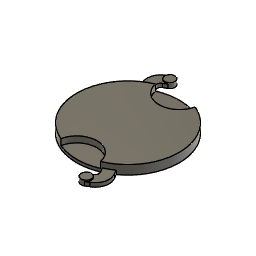
Deckbox - Assembled (Autodesk Fusion 360 archive; units mm, degrees)
design "Deckbox - Key"
Autodesk Fusion 360 part; units mm, degrees
sketch "Sketch1" plane through (0, 0, 0) normal (0, 1, 0) x (1, 0, 0)
  circle A0 centre (0, 0) radius 25.4
  line L0 (19.5918, -28.934) -> (-15.2617, 31.434)
  line L1 (-19.5918, 28.934) -> (15.2617, -31.434)
  line L2 (0, -25.4) -> (0, 25.4) construction
  line L3 (0, 0) -> (25.4, 0) construction
  line L4 (-19.5918, 28.934) -> (-15.2617, 31.434)
  line L5 (15.2617, -31.434) -> (19.5918, -28.934)
  line L6 (17.4268, -30.184) -> (-17.4268, 30.184) construction
  line L7 (-2.1651, -1.25) -> (2.1651, 1.25) construction
  line L8 (19.5918, -28.934) -> (11.7976, -33.434)
  line L9 (11.7976, -33.434) -> (9.2976, -29.1039)
  line L10 (9.2976, -29.1039) -> (17.0918, -24.6039)
  line L11 (17.0918, -24.6039) -> (19.5918, -28.934)
  circle A1 centre (10.5476, -31.269) radius 2.5
  circle A2 centre (0, 0) radius 35.5
  line L12 (-19.5918, 28.934) -> (-17.0918, 24.6039)
  line L13 (-17.0918, 24.6039) -> (-9.2976, 29.1039)
  line L14 (-9.2976, 29.1039) -> (-11.7976, 33.434)
  line L15 (-11.7976, 33.434) -> (-19.5918, 28.934)
  circle A3 centre (-10.5476, 31.269) radius 2.5
  point P0 (-12.5, 21.6506)
  point P1 (12.5, -21.6506)
  dimension "d1" = 50.8
  dimension "d42" = 5
  dimension "d45" = 5
  dimension "d46" = 71
  dimension "d47" = 60
  dimension "d48" = 4
  dimension "d51" = 5
  constraint coincident A0.centre L3.start
  constraint coincident A0 L2.start
  constraint coincident A0 L2.end
  constraint coincident A0.centre L2
  constraint coincident A0 L3.end
  constraint horizontal L3
  constraint perpendicular L0 L4
  constraint perpendicular L0 L5
  constraint perpendicular L1 L4
  constraint midpoint L5 L6.start
  constraint midpoint L4 L6.end
  constraint perpendicular L4 L6
  constraint midpoint L1 L7.start
  constraint midpoint L0 L7.end
  constraint midpoint L6 A0.centre
  constraint perpendicular L8 L9
  constraint parallel L8 L10
  constraint parallel L9 L11
  constraint perpendicular L0 L8
  constraint midpoint L9 A1.centre
  constraint tangent L10 A1
  constraint concentric A0 A2
  constraint tangent A1 A2
  constraint perpendicular L12 L13
  constraint parallel L12 L14
  constraint parallel L13 L15
  constraint coincident L1 L12.end
  constraint midpoint L14 A3.centre
  constraint tangent L13 A3
  constraint tangent A2 A3
  measures "d1" diameter of A0
  measures "d42" distance of L0 L1
  measures "d45" diameter of A1
  measures "d46" diameter of A2 A0.centre
  measures "d47" angle of L3 L6
  measures "d48" distance of L1 A1.centre
  measures "d51" diameter of A3
extrude "Extrude1" add sketch "Sketch1" along normal blind 4.5 contours A0 L0 | A0 L0 L1 | A0 L1
extrude "Extrude2" add sketch "Sketch1" along normal blind 1.9 contours A0 L0 | A0 L0 L1 | A0 L0 L1 L13 | A0 L0 L1 L10 | A0 L1 | L0 L1 L4 L12 L13 L15 | L0 L13 L15 A3 | L0 L1 L5 L8 L10 L11 | L14 A3 | L14 A3 | L1 L8 L10 A1 | L9 A1 | L9 A1
extrude "Extrude3" add sketch "Sketch1" along normal blind 2.5 contours L14 A3 | L14 A3 | L9 A1 | L9 A1
sketch "Sketch2" plane through (0, 4.5, 0) normal (0, 1, 0) x (-1, 0, 0)
  circle A0 centre (0, 0) radius 25.4
  circle A1 centre (0, -25.4) radius 10
  circle A2 centre (0, 25.4) radius 10
  line L0 (0, -25.4) -> (0, 25.4) construction
  dimension "d18" = 20
  dimension "d19" = 20
  constraint coincident A0 A1.centre
  constraint coincident A0 A2.centre
  constraint coincident A1.centre L0.start
  constraint coincident A2.centre L0.end
  constraint coincident A0.centre L0
  constraint vertical L0
  measures "d18" diameter of A1
  measures "d19" diameter of A2
extrude "Extrude4" cut sketch "Sketch2" against normal blind 3 contours A0 A2 | A0 A1 picked at (-1.832, 22.0709) picked at (1.832, -22.0709)
fillet "Fillet6" radius 2 2 edges at (12.7617, 0.95, 27.1039) (-12.7617, 0.95, -27.1039)
fillet "Fillet7" radius 7 2 edges at (19.5918, 0.95, 28.934) (-19.5918, 0.95, -28.934)
named bodies: "Deckbox - Key"

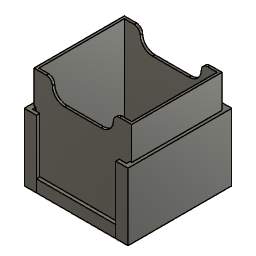
design "Deckbox - Base"
Autodesk Fusion 360 part; units mm, degrees
sketch "Sketch1" plane through (0, 0, 0) normal (0, 1, 0) x (1, 0, 0)
  line L0 (0, 0) -> (76, 0)
  line L1 (76, 0) -> (76, 70)
  line L2 (76, 70) -> (0, 70)
  line L3 (0, 70) -> (0, 0)
  line L4 (-2.25, -2.25) -> (78.25, -2.25)
  line L5 (78.25, -2.25) -> (78.25, 72.25)
  line L6 (78.25, 72.25) -> (-2.25, 72.25)
  line L7 (-2.25, 72.25) -> (-2.25, -2.25)
  line L8 (-0.5, -2.25) -> (76.5, -2.25)
  line L9 (76.5, -2.25) -> (76.5, -4.75)
  line L10 (76.5, -4.75) -> (-0.5, -4.75)
  line L11 (-0.5, -4.75) -> (-0.5, -2.25)
  line L12 (-0.5, -2.25) -> (-4.5, -2.25)
  line L13 (-4.5, -2.25) -> (-4.5, -7.5)
  line L14 (-4.5, -7.5) -> (5.5, -7.5)
  line L15 (5.5, -7.5) -> (5.5, -4.75)
  line L16 (76.5, -2.25) -> (80.5, -2.25)
  line L17 (80.5, -2.25) -> (80.5, -7.5)
  line L18 (80.5, -7.5) -> (70.5, -7.5)
  line L19 (70.5, -7.5) -> (70.5, -4.75)
  line L20 (-4.5, -2.25) -> (80.5, -2.25)
  line L21 (80.5, -2.25) -> (80.5, 77.5)
  line L22 (80.5, 77.5) -> (-4.5, 77.5)
  line L23 (-4.5, 77.5) -> (-4.5, -2.25)
  line L24 (5.5, -7.5) -> (70.5, -7.5)
  point P0 (38, -2.25)
  point P1 (38, -2.25)
  dimension "d3" = 2.25
  dimension "d5" = 2.25
  dimension "d6" = 2.25
  dimension "d7" = 2.25
  dimension "d19" = 77
  dimension "d27" = 10
  dimension "d29" = 5.25
  dimension "d30" = 2.25
  dimension "d58" = 5.25
  dimension "d59" = 2.5
  dimension "d61" = 10
  dimension "d62" = 2.25
  dimension "d77" = 85
  dimension "d78" = 85
  constraint horizontal L0
  constraint vertical L1
  constraint horizontal L2
  constraint vertical L3
  constraint coincident L0.start L3.end
  constraint horizontal L4
  constraint vertical L5
  constraint horizontal L6
  constraint vertical L7
  constraint horizontal L8
  constraint vertical L9
  constraint horizontal L10
  constraint vertical L11
  constraint perpendicular L11 L12
  constraint perpendicular L12 L13
  constraint perpendicular L13 L14
  constraint coincident L10 L15.end
  constraint perpendicular L10 L15
  constraint perpendicular L9 L16
  constraint perpendicular L16 L17
  constraint perpendicular L17 L18
  constraint coincident L10 L19.end
  constraint perpendicular L10 L19
  constraint midpoint L8 P1
  constraint midpoint L4 P1
  constraint coincident P1 P0
  constraint horizontal L20
  constraint vertical L21
  constraint horizontal L22
  constraint vertical L23
  constraint coincident L17 L16.end
  constraint horizontal L24
  measures "d3" distance of L1 L5
  measures "d5" distance of L2 L6
  measures "d6" distance of L3 L7
  measures "d7" distance of L0 L4
  measures "d19" distance of L8.start L8.end
  measures "d27" distance of L17 L19
  measures "d29" distance of L6 L22
  measures "d30" distance of L5 L21
  measures "d58" distance of L4 L24
  measures "d59" distance of L10 L20
  measures "d61" distance of L13 L15
  measures "d62" distance of L7 L23
  measures "d77" distance of L13.end L17.end L0.start
  measures "d78" distance of L13.end L22.end
extrude "Extrude1" add sketch "Sketch1" against normal blind 2 contours L0 L1 L2 L3 | L4 L5 L6 L7 L8 L12 L16 L20 | L5 L6 L7 L12 L16 L20 L21 L22 L23 | L4 L10 L11 L12 L13 L14 L15 L20 | L4 L8 L9 L10 L11 L20 | L4 L9 L10 L16 L17 L18 L19 L20 | L10 L15 L19 L24
extrude "Extrude2" add sketch "Sketch1" along normal blind 80 contours L4 L5 L6 L7 L8 L12 L16 L20
extrude "Extrude3" add sketch "Sketch1" along normal blind 53 contours L5 L6 L7 L12 L16 L20 L21 L22 L23 | L4 L10 L11 L12 L13 L14 L15 L20 | L4 L9 L10 L16 L17 L18 L19 L20
extrude "Extrude5" add sketch "Sketch1" along normal blind 8 contours L10 L15 L19 L24
sketch "Sketch8" plane through (0, 80, 0) normal (0, 1, 0) x (-1, 0, 0)
  line L0 (-78.25, -72.25) -> (2.25, -72.25)
  line L1 (2.25, -72.25) -> (2.25, 2.25)
  line L2 (2.25, 2.25) -> (-78.25, 2.25)
  line L3 (-76, 0) -> (0, 0)
  line L4 (0, 0) -> (0, -70)
  line L5 (0, -70) -> (-76, -70)
  line L6 (2.25, -72.25) -> (-78.25, -72.25)
  line L7 (-78.25, -72.25) -> (-78.25, 2.25)
  line L8 (-78.25, 2.25) -> (2.25, 2.25)
  line L9 (2.25, 2.25) -> (2.25, -72.25)
  line L10 (2, -72) -> (-78, -72)
  line L11 (-78, -72) -> (-78, 2)
  line L12 (-78, 2) -> (2, 2)
  line L13 (2, 2) -> (2, -72)
  line L14 (0.5, 2.25) -> (0.5, 2)
  line L15 (-76.5, 2.25) -> (-76.5, 2)
  line L16 (0.5, 4.75) -> (0.5, 2.25)
  line L17 (-76.5, 2.25) -> (-76.5, 4.75)
  line L18 (-76, -70) -> (-76, 0)
  line L19 (-78.25, 2.25) -> (-78.25, -72.25)
  point P0 (-78.25, 2.25)
  dimension "d80" = 0.25
  dimension "d81" = 0.25
  dimension "d82" = 0.25
  dimension "d83" = 0.25
  constraint horizontal L6
  constraint vertical L7
  constraint horizontal L8
  constraint vertical L9
  constraint coincident L0.end L1.start
  constraint coincident L1.end L2.start
  constraint coincident P0 L2.end
  constraint horizontal L10
  constraint vertical L11
  constraint horizontal L12
  constraint vertical L13
  constraint coincident L12 L14.end
  constraint perpendicular L12 L14
  constraint coincident L12 L15.end
  constraint perpendicular L12 L15
  constraint coincident L8 L14.start
  constraint coincident L14.start L16
  constraint coincident L15.start L17
  measures "d80" distance of L7 L11
  measures "d81" distance of L8 L12
  measures "d82" distance of L9 L13
  measures "d83" distance of L6 L10
extrude "Extrude11" cut sketch "Sketch8" against normal blind 27 contours L0 L1 L2 L6 L7 L8 L9 L10 L11 L12 L13 L14 L15 L19 | L2 L8 L12 L14 L15
extrude "Extrude12" cut sketch "Sketch8" against normal blind 77 contours L2 L8 L12 L14 L15
extrude "Extrude10" add 1 faces at (50.8333, 0, 3.0833) along direction (0, 1, 0) blind 3
sketch "Sketch6" plane through (0, 0, -77.5) normal (0, 0, -1) x (-1, 0, 0)
  circle A0 centre (-38, 53) radius 25.5
  line L0 (4.5, 53) -> (-80.5, 53) construction
  point P0 (-38, 53)
  point P1 (4.5, 53)
  point P2 (-80.5, 53)
  dimension "d40" = 51
  constraint coincident P0 A0.centre
  constraint horizontal L0
  constraint midpoint P0 L0
  constraint coincident P1 L0.start
  constraint coincident P2 L0.end
  measures "d40" diameter of A0
extrude "Extrude7" cut sketch "Sketch6" against normal blind 5.5
sketch "Sketch7" plane through (0, 0, -72) normal (0, 0, -1) x (-1, 0, 0)
  circle A0 centre (-38, 53) radius 35.45
  circle A1 centre (-38, 53) radius 30.25
  circle A2 centre (-38, 53) radius 25.5
  line L0 (-20.5997, 22.8619) -> (-38, 53) construction
  circle A3 centre (-69.45, 53) radius 2.55
  line L1 (-69.45, 53) -> (-38, 53)
  line L2 (-38, 53) -> (-38, 50.45)
  line L3 (-38, 50.45) -> (-69.45, 50.45)
  line L4 (-69.45, 50.45) -> (-69.45, 53)
  line L5 (-40.1651, 51.75) -> (-38, 53)
  line L6 (-20.5997, 22.8619) -> (-22.7648, 21.6119)
  line L7 (-22.7648, 21.6119) -> (-40.1651, 51.75)
  line L8 (-28.8289, 24.1152) -> (-26.2289, 19.6119)
  line L9 (-26.2289, 19.6119) -> (-20.5997, 22.8619)
  circle A4 centre (-27.5289, 21.8635) radius 2.6
  circle A5 centre (-27.7073, 26.9604) radius 2.5
  line L10 (-73.45, 53) -> (-69.45, 53)
  line L11 (-80.5, 53) -> (4.5, 53)
  point P0 (4.5, 53)
  point P1 (-80.5, 53)
  dimension "d52" = 51
  dimension "d55" = 5.1
  dimension "d66" = 4
  dimension "d67" = 5.2
  dimension "d71" = 5
  dimension "d72" = 4
  dimension "d91" = 2.5
  dimension "d92" = 60
  dimension "d93" = 60.5
  constraint concentric A1 A2
  constraint horizontal L1
  constraint vertical L2
  constraint horizontal L3
  constraint vertical L4
  constraint coincident A3.centre L1.start
  constraint parallel L5 L6
  constraint midpoint L8 A4.centre
  constraint tangent A0 A4
  constraint tangent A1 A4
  constraint tangent A4 A5
  constraint tangent A2 A5
  constraint coincident A0 L10.start
  constraint tangent A3 L3
  constraint coincident A0.centre L2
  constraint horizontal L11
  constraint coincident P0 L11.end
  constraint coincident P1 L11.start
  constraint midpoint A0.centre L11
  constraint collinear L1 L11
  constraint collinear L10 L11
  constraint coincident A0.centre A1.centre
  constraint perpendicular L5 L7
  constraint perpendicular L0 L9
  constraint tangent L9 A4
  measures "d52" diameter of A2
  measures "d55" diameter of A3
  measures "d66" distance of L7 L8
  measures "d67" diameter of A4
  measures "d71" diameter of A5
  measures "d72" distance of A3.centre L10.start
  measures "d91" distance of L0 L7
  measures "d92" angle of L0 L11
  measures "d93" diameter of A1
extrude "Extrude8" cut sketch "Sketch7" along normal blind 3.2 contours A0 A1 L7 L9 A4 L11 | L8 A4 | L8 A4 | A1 L7 L9 A4 A5 | A1 A4 A5 | A1 A5
extrude "Extrude9" cut sketch "Sketch7" along normal blind 2.5 contours A0 A1 L7 L9 A4 L11 | L8 A4 | A1 A2 L7 A5 L11 | A3 L4 L10 L11 | L8 A4 | A1 L7 L9 A4 A5 | A1 L7 A5 | A1 A3 L1 L4 L11 | A1 A3 L3 | A1 A3 L1 L11 | A1 A2 A3 L1 L3 L11 | L7 A5 | A2 L1 L3 L5 L7 L11 picked at (-25.3112, 25.8549) picked at (-67.8065, 52.6284)
sketch "Sketch3" plane through (0, 0, 2) normal (0, 0, 1) x (1, 0, 0)
  line L0 (76.5, 3) -> (76.5, 53)
  line L1 (76.5, 53) -> (-0.5, 53)
  line L2 (-0.5, 53) -> (-0.5, 3)
  line L3 (-0.5, 3) -> (76.5, 3)
  line L4 (63, 80) -> (13, 80)
  line L5 (13, 80) -> (13, 65)
  line L6 (13, 65) -> (63, 65)
  line L7 (63, 65) -> (63, 80)
  line L8 (78.25, 80) -> (63, 80)
  line L9 (-2.25, 80) -> (13, 80)
  line L10 (78, 80) -> (-2, 80)
  line L11 (-2, 80) -> (-2, 53)
  line L12 (-2, 53) -> (-0.5, 53)
  line L13 (-0.5, 53) -> (-0.5, 3)
  line L14 (-0.5, 3) -> (76.5, 3)
  line L15 (76.5, 3) -> (76.5, 53)
  line L16 (78, 53) -> (78, 80)
  line L17 (76.5, 53) -> (78, 53)
  dimension "d73" = 15
  dimension "d74" = 50
  constraint horizontal L4
  constraint vertical L5
  constraint horizontal L6
  constraint vertical L7
  constraint equal L8 L9
  measures "d73" distance of L4.start L6.end
  measures "d74" distance of L5.end L6.end
extrude "Extrude4" cut sketch "Sketch3" against normal blind 80 contours L4 L5 L6 L7 L10
fillet "Fillet1" radius 10 6 edges at (13, 65, -71) (13, 65, 1) (13, 65, -71) (63, 65, -71) (63, 65, 1) (63, 65, -71)
fillet "Fillet2" radius 5 5 edges at (63, 80, -71) (63, 80, 1) (13, 80, 1) (13, 80, -71) (13, 80, -71)
named bodies: "Deckbox - Base"

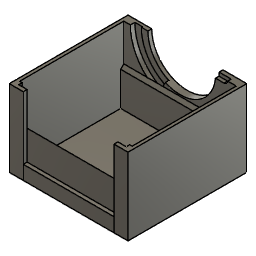
design "Deckbox - Lid"
Autodesk Fusion 360 part; units mm, degrees
sketch "Sketch1" plane through (0, 0, 0) normal (0, 1, 0) x (1, 0, 0)
  line L0 (2.25, 7.5) -> (82.75, 7.5)
  line L1 (82.75, 77.5) -> (2.25, 77.5)
  line L2 (2.25, 5.25) -> (82.75, 5.25)
  line L3 (82.75, 5.25) -> (82.75, 79.75)
  line L4 (82.75, 79.75) -> (2.25, 79.75)
  line L5 (2.25, 79.75) -> (2.25, 5.25)
  line L6 (4, 5.25) -> (81, 5.25)
  line L7 (81, 5.25) -> (81, 2.75)
  line L8 (81, 2.75) -> (4, 2.75)
  line L9 (4, 2.75) -> (4, 5.25)
  line L10 (4, 5.25) -> (0, 5.25)
  line L11 (0, 5.25) -> (0, 0)
  line L12 (0, 0) -> (10, 0)
  line L13 (10, 0) -> (10, 2.75)
  line L14 (81, 5.25) -> (85, 5.25)
  line L15 (85, 5.25) -> (85, 0)
  line L16 (85, 0) -> (75, 0)
  line L17 (75, 0) -> (75, 2.75)
  line L18 (0, 5.25) -> (85, 5.25)
  line L19 (85, 5.25) -> (85, 85)
  line L20 (85, 85) -> (0, 85)
  line L21 (0, 85) -> (0, 5.25)
  line L22 (10, 0) -> (75, 0)
  point P0 (42.5, 5.25)
  point P1 (42.5, 5.25)
  dimension "d5" = 2.25
  dimension "d7" = 2.25
  dimension "d19" = 77
  dimension "d27" = 10
  dimension "d29" = 5.25
  dimension "d30" = 2.25
  dimension "d58" = 5.25
  dimension "d59" = 2.5
  dimension "d61" = 10
  dimension "d62" = 2.25
  dimension "d76" = 85
  dimension "d77" = 85
  constraint horizontal L0
  constraint horizontal L1
  constraint horizontal L2
  constraint vertical L3
  constraint horizontal L4
  constraint vertical L5
  constraint horizontal L6
  constraint vertical L7
  constraint horizontal L8
  constraint vertical L9
  constraint perpendicular L9 L10
  constraint perpendicular L10 L11
  constraint perpendicular L11 L12
  constraint coincident L8 L13.end
  constraint perpendicular L8 L13
  constraint perpendicular L7 L14
  constraint perpendicular L14 L15
  constraint perpendicular L15 L16
  constraint coincident L8 L17.end
  constraint perpendicular L8 L17
  constraint midpoint L6 P1
  constraint midpoint L2 P1
  constraint coincident P1 P0
  constraint horizontal L18
  constraint vertical L19
  constraint horizontal L20
  constraint vertical L21
  constraint coincident L15 L14.end
  constraint horizontal L22
  constraint coincident L1.start L3
  constraint coincident L1.end L5
  constraint coincident L0.start L5
  constraint coincident L0.end L3
  constraint coincident L11.end L12.start
  measures "d5" distance of L1 L4
  measures "d7" distance of L0 L2
  measures "d19" distance of L6.start L6.end
  measures "d27" distance of L15 L17
  measures "d29" distance of L4 L20
  measures "d30" distance of L3 L19
  measures "d58" distance of L2 L22
  measures "d59" distance of L8 L18
  measures "d61" distance of L11 L13
  measures "d62" distance of L5 L21
  measures "d76" distance of L11.end L15.end
  measures "d77" distance of L11.end L20.end
extrude "Extrude1" add sketch "Sketch1" against normal blind 2
extrude "Extrude2" add sketch "Sketch1" along normal blind 26.5 contours L0 L2 L3 L5 L6 L10 L14 L18 | L1 L3 L4 L5
extrude "Extrude3" add sketch "Sketch1" along normal blind 53 contours L3 L4 L5 L10 L14 L18 L19 L20 L21 | L2 L8 L9 L10 L11 L12 L13 L18 | L2 L7 L8 L14 L15 L16 L17 L18
extrude "Extrude5" add sketch "Sketch1" along normal blind 8 contours L8 L13 L17 L22
extrude "Extrude10" add 1 faces at (55.3333, 0, -4.4167) along direction (0, 1, 0) blind 3
sketch "Sketch6" plane through (0, 0, -85) normal (0, 0, -1) x (-1, 0, 0)
  circle A0 centre (-42.5, 53) radius 25.5
  line L0 (0, 53) -> (-85, 53) construction
  point P0 (-42.5, 53)
  point P1 (0, 53)
  point P2 (-85, 53)
  dimension "d40" = 51
  constraint coincident P0 A0.centre
  constraint horizontal L0
  constraint midpoint P0 L0
  constraint coincident P1 L0.start
  constraint coincident P2 L0.end
  measures "d40" diameter of A0
extrude "Extrude7" cut sketch "Sketch6" against normal blind 5.25
sketch "Sketch7" plane through (0, 0, -85) normal (0, 0, -1) x (-1, 0, 0)
  circle A0 centre (-42.5, 53) radius 35.55
  circle A1 centre (-42.5, 53) radius 30.25
  circle A2 centre (-42.5, 53) radius 25.5
  line L0 (-26.4898, 25.2696) -> (-42.5, 53) construction
  circle A3 centre (-74.05, 53) radius 2.55
  line L1 (-74.05, 53) -> (-42.5, 53)
  line L2 (-42.5, 53) -> (-42.5, 50.45)
  line L3 (-42.5, 50.45) -> (-74.05, 50.45)
  line L4 (-74.05, 50.45) -> (-74.05, 53)
  line L5 (-44.6651, 51.75) -> (-42.5, 53)
  line L6 (-26.4898, 25.2696) -> (-28.6549, 24.0196)
  line L7 (-28.6549, 24.0196) -> (-44.6651, 51.75)
  circle A4 centre (-33.0344, 21.4911) radius 2.65
  circle A5 centre (-33.0551, 26.641) radius 2.5
  line L8 (-78.05, 53) -> (-74.05, 53)
  line L9 (-28.6549, 24.0196) -> (-33.0344, 21.4911)
  line L10 (-85, 53) -> (0, 53)
  point P0 (-85, 53)
  point P1 (0, 53)
  dimension "d52" = 51
  dimension "d55" = 5.1
  dimension "d67" = 5.3
  dimension "d71" = 5
  dimension "d72" = 4
  dimension "d81" = 2.5
  dimension "d82" = 60
  dimension "d85" = 60.5
  constraint horizontal L1
  constraint vertical L2
  constraint horizontal L3
  constraint vertical L4
  constraint coincident A3.centre L1.start
  constraint parallel L5 L6
  constraint tangent A0 A4
  constraint tangent A1 A4
  constraint tangent A4 A5
  constraint tangent L7 A5
  constraint tangent A2 A5
  constraint coincident A0 L8.start
  constraint tangent A3 L3
  constraint coincident A0.centre L2
  constraint coincident L0.start L6.start
  constraint perpendicular L0 L6
  constraint coincident A0.centre A1.centre
  constraint perpendicular L7 L9
  constraint coincident A4.centre L9.end
  constraint coincident P0 L10.start
  constraint coincident P1 L10.end
  constraint midpoint A0.centre L10
  constraint collinear L8 L10
  measures "d52" diameter of A2
  measures "d55" diameter of A3
  measures "d67" diameter of A4
  measures "d71" diameter of A5
  measures "d72" distance of A3.centre L8.start
  measures "d81" distance of L0 L7
  measures "d82" angle of L0 L10
  measures "d85" diameter of A1
extrude "Extrude8" cut sketch "Sketch7" along normal blind 3.2 from surface at -5.25 contours A0 A1 L7 A4 L9 L10 | A4 | A1 A4 A5 | A1 L7 A4 A5 L9 | A1 A5 picked at (-32.2182, 24.4659)
extrude "Extrude9" cut sketch "Sketch7" along normal blind 2.5 from surface at -5.25 contours A0 A1 L7 A4 L9 L10 | A1 A2 L7 L10 | A3 L4 L8 L10 | A1 A3 L1 L8 L10 | A1 A3 L1 L10 | A1 L7 A5 | A1 A3 L1 L4 L10 | A1 A3 L3 | A1 A2 A3 L1 L3 L10 | A1 A3 L1 L10 | A2 L1 L3 L5 L7 L10 | L2 L3 L5 L7
extrude "Extrude11" cut 1 faces at (55.3333, 3, -4.4167) along direction (0, -1, 0) blind 3
sketch "Sketch8" plane through (0, 26.5, 0) normal (0, 1, 0) x (-1, 0, 0)
  line L0 (-2.25, -79.75) -> (-2.25, -77.5)
  line L1 (-2.25, -5.25) -> (-4, -5.25)
  line L2 (-4, -5.25) -> (-81, -5.25)
  line L3 (-81, -5.25) -> (-82.75, -5.25)
  line L4 (-82.75, -77.5) -> (-82.75, -79.75)
  line L5 (-82.75, -79.75) -> (-30.5591, -79.75)
  line L6 (-30.5591, -79.75) -> (-18.8029, -79.75)
  line L7 (-4, -5.25) -> (-81, -5.25)
  line L8 (-81, -5.25) -> (-81, -5.5)
  line L9 (-81, -5.5) -> (-4, -5.5)
  line L10 (-4, -5.5) -> (-4, -5.25)
  line L11 (-18.8029, -79.75) -> (-2.25, -79.75)
  line L12 (-2.25, -77.5) -> (-82.75, -77.5)
  line L13 (-2.25, -7.5) -> (-2.25, -5.25)
  line L14 (-82.75, -5.25) -> (-82.75, -7.5)
  line L15 (-82.75, -7.5) -> (-2.25, -7.5)
  dimension "d78" = 0.25
  constraint horizontal L7
  constraint vertical L8
  constraint horizontal L9
  constraint vertical L10
  constraint coincident L1.end L2.start
  constraint coincident L2.end L8
  measures "d78" distance of L7 L9
extrude "Extrude12" cut sketch "Sketch8" against normal blind 26 contours L2 L7 L8 L9 L10
chamfer "Chamfer2" distance 2.25 angle 45 2 edges at (42.5, 26.5, -77.5) (42.5, 26.5, -7.5)
equation "d69 = 0 mm - 5.25 mm"
named bodies: "Deckbox - Lid"
